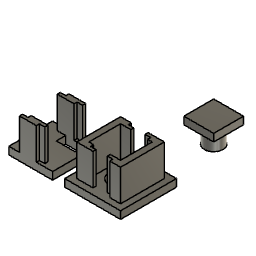
button (Autodesk Fusion 360 design; units mm, degrees)
Autodesk Fusion 360 part; units mm, degrees
sketch "Sketch1" plane through (0, 0, 0) normal (0, 0, 1) x (1, 0, 0)
  line L0 (0, 0) -> (15, 0)
  line L1 (15, 0) -> (15, 15)
  line L2 (15, 15) -> (0, 15)
  line L3 (0, 15) -> (0, 0)
  line L4 (3.25, 11.75) -> (11.75, 11.75)
  line L5 (11.75, 11.75) -> (11.75, 3.25)
  line L6 (11.75, 3.25) -> (3.25, 3.25)
  line L7 (3.25, 3.25) -> (3.25, 11.75)
  line L8 (1.625, 13.375) -> (13.375, 13.375)
  line L9 (13.375, 13.375) -> (13.375, 1.625)
  line L10 (13.375, 1.625) -> (1.625, 1.625)
  line L11 (1.625, 1.625) -> (1.625, 13.375)
  circle A0 centre (7.5, 7.5) radius 3
  dimension "d1" = 15
  dimension "d2" = 15
  dimension "d3" = 8.5
  dimension "d4" = 8.5
  dimension "d5" = 3.25
  dimension "d6" = 3.25
  dimension "d7" = 1.625
  dimension "d8" = 1.625
  dimension "d9" = 1.625
  dimension "d10" = 1.625
  dimension "d15" = 6
  dimension "d16" = 4.25
  dimension "d17" = 4.25
  constraint horizontal L0
  constraint vertical L1
  constraint horizontal L2
  constraint vertical L3
  constraint coincident L0.start L3.end
  constraint horizontal L4
  constraint vertical L5
  constraint horizontal L6
  constraint vertical L7
  constraint horizontal L8
  constraint vertical L9
  constraint horizontal L10
  constraint vertical L11
  measures "d1" distance of L0.start L0.end
  measures "d2" distance of L0.start L2.end
  measures "d3" distance of L4.start L4.end
  measures "d4" distance of L4.start L6.end
  measures "d5" distance of L0 L6
  measures "d6" distance of L3 L7
  measures "d7" distance of L5 L9
  measures "d8" distance of L4 L8
  measures "d9" distance of L7 L11
  measures "d10" distance of L6 L10
  measures "d15" diameter of A0
  measures "d16" distance of L5 A0.centre
  measures "d17" distance of L6 A0.centre
extrude "Extrude1" add sketch "Sketch1" along normal blind 2 contours L0 L1 L2 L3 | L4 L5 L6 L7 | A0 makes body 1 at (6.0833, 8.9167, 0) makes body 2 at (5.5417, 0.5417, 0)
extrude "Extrude2" add sketch "Sketch1" along normal blind 10.5 contours L8 L9 L10 L11 bodies 1 2
extrude "Extrude3" cut sketch "Sketch1" along normal blind 2 contours A0 bodies 1
sketch "Sketch2" plane through (0, 0, 10.5) normal (0, 0, 1) x (-1, 0, 0)
  line L0 (-11.75, -3.25) -> (-3.25, -3.25)
  line L1 (-3.25, -3.25) -> (-3.25, -11.75)
  line L2 (-3.25, -11.75) -> (-11.75, -11.75)
  line L3 (-11.75, -11.75) -> (-11.75, -3.25)
  line L4 (-1.625, -1.625) -> (-13.375, -1.625)
  line L5 (-13.375, -1.625) -> (-13.375, -13.375)
  line L6 (-13.375, -13.375) -> (-1.625, -13.375)
  line L7 (-1.625, -13.375) -> (-1.625, -1.625)
  line L8 (-7.5, -13.375) -> (-9, -13.375)
  line L9 (-9, -13.375) -> (-9, -11.75)
  line L10 (-9, -11.75) -> (-7.5, -11.75)
  line L11 (-7.5, -11.75) -> (-7.5, -13.375)
  line L12 (-7.5, -13.375) -> (-6, -13.375)
  line L13 (-6, -13.375) -> (-6, -11.75)
  line L14 (-6, -11.75) -> (-7.5, -11.75)
  line L15 (-7.5, -11.75) -> (-7.5, -13.375)
  line L16 (-7.5, -3.25) -> (-9, -3.25)
  line L17 (-9, -3.25) -> (-9, -1.625)
  line L18 (-9, -1.625) -> (-7.5, -1.625)
  line L19 (-7.5, -1.625) -> (-7.5, -3.25)
  line L20 (-7.5, -3.25) -> (-6, -3.25)
  line L21 (-6, -3.25) -> (-6, -1.625)
  line L22 (-6, -1.625) -> (-7.5, -1.625)
  line L23 (-7.5, -1.625) -> (-7.5, -3.25)
  dimension "d20" = 1.5
  dimension "d21" = 1.5
  constraint horizontal L8
  constraint vertical L9
  constraint horizontal L10
  constraint vertical L11
  constraint midpoint L6 L8.start
  constraint horizontal L12
  constraint vertical L13
  constraint horizontal L14
  constraint vertical L15
  constraint horizontal L16
  constraint vertical L17
  constraint horizontal L18
  constraint vertical L19
  constraint midpoint L0 L16.start
  constraint horizontal L20
  constraint vertical L21
  constraint horizontal L22
  constraint vertical L23
  measures "d20" distance of L8.start L8.end
  measures "d21" distance of L16.start L16.end
extrude "Extrude4" cut sketch "Sketch2" against normal blind 8.5 contours L0 L4 L16 L17 L18 L19 L23 | L0 L4 L19 L20 L21 L22 L23 | L2 L6 L8 L9 L10 L11 L15 | L2 L6 L11 L12 L13 L14 L15 bodies 1
sketch "Sketch3" plane through (6, 0, 0) normal (1, 0, 0) x (0, 1, 0)
  line L0 (3.25, 10.5) -> (1.625, 10.5)
  line L1 (1.625, 10.5) -> (1.625, 2)
  line L2 (1.625, 2) -> (3.25, 2)
  line L3 (3.25, 2) -> (3.25, 10.5)
  line L4 (3.25, 10.5) -> (2.4375, 10.5)
  line L5 (2.4375, 10.5) -> (2.4375, 2)
  line L6 (2.4375, 2) -> (3.25, 2)
  line L7 (3.25, 2) -> (3.25, 10.5)
  line L8 (13.375, 10.5) -> (12.562, 10.5)
  line L9 (12.562, 10.5) -> (12.562, 2)
  line L10 (12.562, 2) -> (13.375, 2)
  line L11 (13.375, 2) -> (13.375, 10.5)
  dimension "d24" = 0.8125
  dimension "d25" = 8.5
  dimension "d26" = 0.813
  dimension "d27" = 8.5
  constraint horizontal L4
  constraint vertical L5
  constraint horizontal L6
  constraint vertical L7
  constraint coincident L0.start L3.end
  constraint horizontal L8
  constraint vertical L9
  constraint horizontal L10
  constraint vertical L11
  measures "d24" distance of L0.start L4.end
  measures "d25" distance of L0.start L2.end
  measures "d26" distance of L8.start L8.end
  measures "d27" distance of L8.start L10.end
extrude "Extrude5" cut sketch "Sketch3" against normal blind 1.5 contours L0 L2 L3 L4 L5 L6 L7 | L8 L9 L10 L11 bodies 1
sketch "Sketch4" plane through (9, 0, 0) normal (-1, 0, 0) x (0, -1, 0)
  line L0 (-11.75, 10.5) -> (-13.375, 10.5)
  line L1 (-13.375, 10.5) -> (-13.375, 2)
  line L2 (-13.375, 2) -> (-11.75, 2)
  line L3 (-11.75, 2) -> (-11.75, 10.5)
  line L4 (-11.75, 10.5) -> (-12.5625, 10.5)
  line L5 (-12.5625, 10.5) -> (-12.5625, 2)
  line L6 (-12.5625, 2) -> (-11.75, 2)
  line L7 (-11.75, 2) -> (-11.75, 10.5)
  line L8 (-1.625, 10.5) -> (-2.438, 10.5)
  line L9 (-2.438, 10.5) -> (-2.438, 2)
  line L10 (-2.438, 2) -> (-1.625, 2)
  line L11 (-1.625, 2) -> (-1.625, 10.5)
  dimension "d30" = 8.5
  dimension "d31" = 0.813
  dimension "d32" = 8.5
  constraint horizontal L4
  constraint vertical L5
  constraint horizontal L6
  constraint vertical L7
  constraint coincident L0.start L3.end
  constraint horizontal L8
  constraint vertical L9
  constraint horizontal L10
  constraint vertical L11
  measures "d30" distance of L0.start L2.end
  measures "d31" distance of L8.start L8.end
  measures "d32" distance of L8.start L10.end
extrude "Extrude6" cut sketch "Sketch4" against normal blind 1.5 contours L0 L2 L3 L4 L5 L6 L7 | L8 L9 L10 L11 bodies 1
sketch "Sketch5" plane through (0, 0, 0) normal (0, 0, 1) x (1, 0, 0)
  line L0 (-15, 0) -> (-3.25, 0)
  line L1 (-3.25, 0) -> (-3.25, 11.75)
  line L2 (-3.25, 11.75) -> (-15, 11.75)
  line L3 (-15, 11.75) -> (-15, 0)
  line L4 (-10.625, 11.75) -> (-6.125, 11.75)
  line L5 (-6.125, 11.75) -> (-6.125, 10.937)
  line L6 (-6.125, 10.937) -> (-10.625, 10.937)
  line L7 (-10.625, 10.937) -> (-10.625, 11.75)
  line L8 (-12.125, 10.937) -> (-7.625, 10.937)
  line L9 (-7.625, 10.937) -> (-7.625, 10.124)
  line L10 (-7.625, 10.124) -> (-12.125, 10.124)
  line L11 (-12.125, 10.124) -> (-12.125, 10.937)
  line L12 (-12.125, 0) -> (-7.625, 0)
  line L13 (-7.625, 0) -> (-7.625, 0.813)
  line L14 (-7.625, 0.813) -> (-12.125, 0.813)
  line L15 (-12.125, 0.813) -> (-12.125, 0)
  line L16 (-6.125, 0.813) -> (-10.625, 0.813)
  line L17 (-10.625, 0.813) -> (-10.625, 1.643)
  line L18 (-10.625, 1.643) -> (-6.125, 1.643)
  line L19 (-6.125, 1.643) -> (-6.125, 0.813)
  line L20 (-9.875, 10.124) -> (-4.875, 10.124)
  line L21 (-4.875, 10.124) -> (-4.875, 7.624)
  line L22 (-4.875, 7.624) -> (-9.875, 7.624)
  line L23 (-9.875, 7.624) -> (-9.875, 10.124)
  dimension "d35" = 11.75
  dimension "d36" = 11.75
  dimension "d38" = 2.875
  dimension "d39" = 0.813
  dimension "d40" = 4.5
  dimension "d41" = 0.813
  dimension "d42" = 4.375
  dimension "d43" = 4.5
  dimension "d44" = 0.813
  dimension "d45" = 4.375
  dimension "d46" = 4.5
  dimension "d47" = 0.83
  dimension "d48" = 2.875
  dimension "d49" = 5
  dimension "d50" = 2.5
  dimension "d51" = 1.625
  dimension "d52" = 4.5
  constraint horizontal L0
  constraint vertical L1
  constraint horizontal L2
  constraint vertical L3
  constraint horizontal L4
  constraint vertical L5
  constraint horizontal L6
  constraint vertical L7
  constraint coincident L2 L4.start
  constraint horizontal L8
  constraint vertical L9
  constraint horizontal L10
  constraint vertical L11
  constraint coincident L6 L8.start
  constraint horizontal L12
  constraint vertical L13
  constraint horizontal L14
  constraint vertical L15
  constraint coincident L0 L12.start
  constraint horizontal L16
  constraint vertical L17
  constraint horizontal L18
  constraint vertical L19
  constraint coincident L14 L16.start
  constraint horizontal L20
  constraint vertical L21
  constraint horizontal L22
  constraint vertical L23
  constraint coincident L10 L20.start
  measures "d35" distance of L0.start L0.end
  measures "d36" distance of L0.start L2.end
  measures "d38" distance of L1 L5
  measures "d39" distance of L2 L6
  measures "d40" distance of L8.start L8.end
  measures "d41" distance of L8.start L10.end
  measures "d42" distance of L1 L9
  measures "d43" distance of L12.start L12.end
  measures "d44" distance of L12.start L14.end
  measures "d45" distance of L1 L13
  measures "d46" distance of L16.start L16.end
  measures "d47" distance of L16.start L18.end
  measures "d48" distance of L1 L19
  measures "d49" distance of L20.start L20.end
  measures "d50" distance of L20.start L22.end
  measures "d51" distance of L1 L21
  measures "d52" distance of L5.end L6.end
extrude "Extrude7" add sketch "Sketch5" along normal blind 10.5 separate body contours L0 L12 L13 L14 L15 L16 | L2 L4 L5 L6 L7 L8 | L14 L16 L17 L18 L19 | L6 L8 L9 L10 L11 L20 makes body 3 at (-7.625, 11.75, 3.5) makes body 4 at (-10.625, 0, 3.5)
extrude "Extrude8" add sketch "Sketch5" along normal blind 2 contours L0 L1 L2 L3 L5 L6 L7 L8 L9 L10 L11 L13 L14 L15 L16 L17 L18 L19 L20 L21 L22 L23 bodies 3 4
sketch "Sketch6" plane through (0, 0, 0) normal (0, 0, 1) x (1, 0, 0)
  circle A0 centre (10, 30) radius 2.5
  line L0 (9, 31.5) -> (11, 31.5)
  line L1 (11, 31.5) -> (11, 28.5)
  line L2 (11, 28.5) -> (9, 28.5)
  line L3 (9, 28.5) -> (9, 31.5)
  dimension "d57" = 5
  dimension "d58" = 2
  dimension "d59" = 3
  dimension "d60" = 1
  dimension "d61" = 1.5
  constraint horizontal L0
  constraint vertical L1
  constraint horizontal L2
  constraint vertical L3
  measures "d57" diameter of A0
  measures "d58" distance of L0.start L0.end
  measures "d59" distance of L0.start L2.end
  measures "d60" distance of A0.centre L1
  measures "d61" distance of A0.centre L0
extrude "Extrude9" add sketch "Sketch6" along normal blind 2.5 separate body makes body 5
sketch "Sketch7" plane through (0, 0, 2.5) normal (0, 0, 1) x (-1, 0, 0)
  line L0 (-11, -28.5) -> (-9, -28.5)
  line L1 (-9, -28.5) -> (-9, -31.5)
  line L2 (-9, -31.5) -> (-11, -31.5)
  line L3 (-11, -31.5) -> (-11, -28.5)
  circle A0 centre (-10, -30) radius 2.5
  circle A1 centre (-10, -30) radius 2.5
  constraint concentric A0 A1
extrude "Extrude10" add sketch "Sketch7" along normal blind 2 contours L0 L1 L2 L3 | A0 A1 bodies 5
sketch "Sketch8" plane through (0, 0, 4.5) normal (0, 0, 1) x (-1, 0, 0)
  circle A0 centre (-10, -30) radius 2.5
  line L0 (-10, -30) -> (-14, -30)
  line L1 (-14, -30) -> (-14, -26)
  line L2 (-14, -26) -> (-10, -26)
  line L3 (-10, -26) -> (-10, -30)
  line L4 (-10, -30) -> (-6, -30)
  line L5 (-6, -30) -> (-6, -34)
  line L6 (-6, -34) -> (-10, -34)
  line L7 (-10, -34) -> (-10, -30)
  line L8 (-6, -34) -> (-14, -34)
  line L9 (-14, -34) -> (-14, -26)
  line L10 (-14, -26) -> (-6, -26)
  line L11 (-6, -26) -> (-6, -34)
  dimension "d66" = 4
  dimension "d67" = 4
  dimension "d68" = 4
  dimension "d69" = 4
  constraint horizontal L0
  constraint vertical L1
  constraint horizontal L2
  constraint vertical L3
  constraint coincident A0.centre L0.start
  constraint horizontal L4
  constraint vertical L5
  constraint horizontal L6
  constraint vertical L7
  constraint horizontal L8
  constraint vertical L9
  constraint horizontal L10
  constraint vertical L11
  measures "d66" distance of A0.centre L0.end
  measures "d67" distance of A0.centre L2.end
  measures "d68" distance of A0.centre L6.end
  measures "d69" distance of L5.end L6.end
extrude "Extrude11" add sketch "Sketch8" along normal blind 2 bodies 5
equation "d7 = ( 3.25 / 2 ) * 1 mm"
equation "d8 = ( 3.25 / 2 ) * 1 mm"
equation "d16 = ( 8.5 / 2 ) * 1 mm"
equation "d24 = ( 1.625 / 2 ) * 1 mm"
